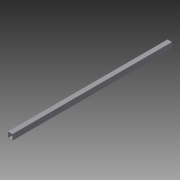
# Autodesk Inventor part: Part1
Saved by Autodesk Inventor 2015 SP1 (Build 190203100, 203)
## iProperties
Created: 2015-03-28
Part Number: Part1
Material: Generic
Document SubType Name: Modeling
Designer: Cyril
Density: 1 g/cm^3
Appearance: Default
Author: Cyril
Autodesk Inventor part; units mm, degrees
ref_plane "YZ Plane" through (0, 0, 0) normal (1, 0, 0) x (0, 1, 0)
ref_plane "XZ Plane" through (0, 0, 0) normal (0, 1, 0) x (-1, 0, 0)
ref_plane "XY Plane" through (0, 0, 0) normal (0, 0, 1) x (1, 0, 0)
sketch "Sketch2" plane through (0, 0, 0) normal (0, 0, 1) x (1, 0, 0)
  line L0 (-18, -23) -> (18, -23)
  line L1 (18, -23) -> (18, 23)
  line L2 (18, 23) -> (-18, 23)
  line L3 (-18, 23) -> (-18, -23)
  line L4 (-18, -22.5) -> (18, 22.5) construction
  line L5 (18, -23) -> (-15.1101, 19.3073) construction
  line L6 (-20, -25) -> (20, -25)
  line L7 (20, -25) -> (20, 25)
  line L8 (20, 25) -> (-20, 25)
  line L9 (-20, 25) -> (-20, -25)
  line L10 (-20, -25) -> (20, 25) construction
  line L11 (20, -25) -> (-20, 25) construction
  point P0 (0, 0)
  dimension "d0" = 40
  dimension "d1" = 50
  dimension "d3" = 2
  dimension "d6" = 2
  dimension "d7" = 2
  dimension "d8" = 2
  constraints: 24 end point, 4 parallel, 3 midpoint, 2 horizontal, 2 perpendicular, 2 point on line
  measures "d0" distance of L7.end L8.end
  measures "d1" distance of L8.end L6.start
  measures "d3" distance between parallel lines of L9 L3
  measures "d6" distance between parallel lines of L8 L2
  measures "d7" distance between parallel lines of L7 L1
  measures "d8" distance between parallel lines of L6 L0
extrude "Extrusion1" add sketch "Sketch2" along normal mid plane 1430
equation "\"d6\" = d3"
equation "\"d7\" = d3"
body "Solid1"
